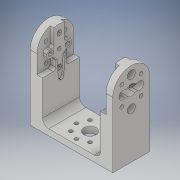
# Autodesk Inventor part: Module_Arm
Saved by Autodesk Inventor 2018 (Build 220112000, 112)
## iProperties
Created: 2016-10-25
Part Number: Module_Arm
Material: Generic
Document SubType Name: Modeling
Designer: Lucas
Density: 1 g/cm^3
Appearance: Default
Author: Lucas
Autodesk Inventor part; units mm, degrees
ref_plane "YZ Plane" through (0, 0, 0) normal (1, 0, 0) x (0, 1, 0)
sketch "Sketch1" plane through (0, 0, 0) normal (0, 0, 1) x (1, 0, 0)
  line L0 (0, 0) -> (47, 0)
  line L1 (47, 0) -> (47, 63)
  line L2 (47, 63) -> (57, 63)
  line L3 (57, 63) -> (57, -5)
  line L4 (57, -5) -> (-10, -5)
  line L5 (-10, -5) -> (-10, 63)
  line L6 (-10, 63) -> (0, 63)
  line L7 (0, 63) -> (0, 0)
  dimension "d0" = 47
  dimension "d1" = 63
  dimension "d2" = 10
  dimension "d13" = 5
  dimension "d64" = 10
  constraints: 16 end point, 5 perpendicular, 2 point on line, 1 horizontal, 1 vertical
  measures "d0" distance of L0.start L0.end
  measures "d1" distance of L0.end L1.end
  measures "d2" distance of L1.end L2.end
  measures "d13" distance between parallel lines of L4 L0
  measures "d64" distance of L5.end L6.end
extrude "U_Profile" add sketch "Sketch1" along normal blind 30
sketch "Sketch2" plane through (57, -5, 0) normal (1, 0, 0) x (0, 0, -1)
  circle A0 centre (-15, 50.6) radius 1.5
  line L0 (-15, 55.5625) -> (-15, -8.8186) construction
  line L1 (-30, 0) -> (-30, 68) projected
  line L2 (0, 68) -> (0, 0) projected
  line L3 (0, 68) -> (-30, 68) projected
  point P0 (0, 5)
  dimension "d7" = 3
  dimension "d8" = 30
  dimension "d9" = 15
  dimension "d10" = 17.4
  constraints: 2 end point, 1 centre point, 1 point on line, 1 vertical
  measures "d7" diameter of A0
  measures "d8" distance between parallel lines of L1 L2
  measures "d9" distance between parallel lines of L0 L2
  measures "d10" distance from line of A0.centre L3
extrude "Shaft_Opening" cut sketch "Sketch2" against normal up to surface (67 mm away)
sketch "Sketch4" plane through (-10, -5, 0) normal (-1, 0, 0) x (0, 0, 1)
  circle A0 centre (15, 50.6) radius 5
  circle A1 centre (15, 50.6) radius 1.5 projected
  point P0 (0, 5)
  dimension "d18" = 10
  constraints: 1 centre point, 1 concentric
  measures "d18" diameter of A0
extrude "Nut_Slot" cut sketch "Sketch4" against normal blind 5.5
sketch "Sketch6" plane through (0, 0, 0) normal (0, 1, 0) x (1, 0, 0)
  circle A0 centre (23.5, -15) radius 11 construction
  line L0 (0, -15) -> (46.0375, -15)
  line L1 (47, -30) -> (0, -30) projected
  line L2 (0, 0) -> (47, 0) projected
  line L3 (0, 0) -> (0, -30) projected
  line L4 (47, 0) -> (47, -30) projected
  circle A1 centre (12.5, -15) radius 1.5
  circle A2 centre (34.5, -15) radius 1.5
  line L5 (9.9716, -1.4716) -> (37.7642, -29.2642) construction
  line L6 (9.808, -28.692) -> (35.7154, -2.7846) construction
  line L7 (23.5, 2.3185) -> (23.5, -31.0285) construction
  circle A3 centre (15.7218, -7.2218) radius 1.5
  circle A4 centre (23.5, -4) radius 1.5
  circle A5 centre (31.2782, -7.2218) radius 1.5
  circle A6 centre (23.5, -26) radius 1.5
  circle A7 centre (15.7218, -22.7782) radius 1.5
  circle A8 centre (31.2782, -22.7782) radius 1.5
  dimension "d21" = 22
  dimension "d22" = 30
  dimension "d23" = 15
  dimension "d24" = 23.5
  dimension "d25" = 47
  dimension "d26" = 3
  dimension "d27" = 3
  dimension "d28" = 45
  dimension "d29" = 45
  dimension "d30" = 90
  dimension "d31" = 3
  dimension "d32" = 3
  dimension "d33" = 3
  dimension "d34" = 3
  dimension "d35" = 3
  dimension "d36" = 3
  constraints: 12 point on line, 8 centre point, 8 end point, 1 horizontal, 10 other
  measures "d22" distance between parallel lines of L1 L2
  measures "d23" distance between parallel lines of L2 L0
  measures "d24" distance from line of point (23.5, -15) L3
  measures "d25" distance between parallel lines of L4 L3
  measures "d26" diameter of A1
  measures "d27" diameter of A2
  measures "d28" angle of L5 L0
  measures "d29" angle of L0 L6
  measures "d30" angle of L0 L7
  measures "d31" diameter of A3
  measures "d32" diameter of A4
  measures "d33" diameter of A5
  measures "d34" diameter of A6
  measures "d35" diameter of A7
  measures "d36" diameter of A8
extrude "Docking_Holes_Front" cut sketch "Sketch6" against normal up to surface (5 mm away) contours A1 L0 | L0 A1 | A2 L0 | L0 A2 | A3 | A4 | A5 | A6 | A7 | A8
sketch "Sketch8" plane through (47, 0, 4) normal (-1, 0, 0) x (0, 0, 1)
  line L0 (19.4554, 45.6) -> (2.5446, 45.6) construction
  line L1 (11, 58.3863) -> (11, 17.922) construction
  line L2 (13, 24.6021) -> (9, 24.6021) construction
  line L3 (14.5, 43.6) -> (12.9998, 24.6)
  line L4 (7.5, 43.6) -> (9, 24.6021)
  line L5 (19.4554, 45.6) -> (13.9554, 45.6) construction
  line L6 (2.5446, 45.6) -> (8.0446, 45.6) construction
  line L7 (13, 58.6) -> (9, 58.6) construction
  line L8 (13.9554, 45.6) -> (12.7795, 61.6) construction
  line L9 (8.0446, 45.6) -> (9.2205, 61.6) construction
  line L10 (12.7795, 61.6) -> (9.2205, 61.6) construction
  line L11 (12.9998, 24.6) -> (9, 24.6021)
  line L12 (7.5, 43.6) -> (-4, 43.6)
  line L13 (14.5, 43.6) -> (26, 43.6)
  line L14 (-4, 0) -> (-4, 63) projected
  line L15 (-4, 43.6) -> (-4, 63)
  line L16 (-4, 63) -> (26, 63) projected
  line L17 (-4, 63) -> (26, 63)
  line L18 (26, 63) -> (26, 43.6)
  point P0 (11, 45.6)
  dimension "d48" = 4
  dimension "d52" = 19
  dimension "d54" = 5.5
  dimension "d55" = 5.5
  dimension "d56" = 4
  dimension "d57" = 13
  dimension "d58" = 16
  dimension "d59" = 16
  dimension "d109" = 2
  dimension "d183" = 2
  dimension "d189" = 3.9998
  dimension "d221" = 2
  dimension "d256" = 15
  dimension "d257" = 3.5
  constraints: 34 end point, 7 point on line, 4 horizontal, 2 collinear, 2 symmetric about line, 1 midpoint, 1 parallel, 1 perpendicular, 1 vertical, 1 other
  measures "d48" distance of L2.start L2.end
  measures "d52" vertical distance of L3.start L3.end
  measures "d54" distance of L0.start L5.end
  measures "d55" distance of L0.end L6.end
  measures "d56" distance of L7.start L7.end
  measures "d57" distance between parallel lines of L0 L7
  measures "d58" vertical distance of L5.end L8.end
  measures "d59" vertical distance of L6.end L9.end
  measures "d109" distance from line of L1 L4.end
  measures "d183" distance between parallel lines of L13 L0
  measures "d189" distance of L3.end L4.end
  measures "d221" distance from line of L12 point (11, 45.6)
  measures "d256" distance between parallel lines of L15 L1
  measures "d257" distance from line of L4.start L1
extrude "Servo_Horn_Slot" cut sketch "Sketch8" against normal blind 1.5
fillet "Fillet4" radius 2 2 edges at (47.75, 24.6021, 13) (47.75, 24.6, 16.9998)
fillet "Fillet9" radius 15 4 edges at (-5, 63, 0) (-5, 63, 30) (52.75, 63, 0) (52.75, 63, 30)
sketch "Sketch11" plane through (-10, -5, 0) normal (-1, 0, 0) x (0, 0, 1)
  circle A0 centre (15, 50.6) radius 11 construction
  circle A1 centre (15, 50.6) radius 1.5 projected
  line L0 (1.3636, 36.9636) -> (45.6005, 81.2005) construction
  line L1 (1.3398, 64.2602) -> (31.9798, 33.6202) construction
  line L2 (15, 20.4128) -> (15, 77.5107)
  circle A2 centre (7.2218, 42.8218) radius 1.5
  circle A3 centre (7.2218, 58.3782) radius 1.5
  circle A4 centre (22.7782, 42.8218) radius 1.5
  circle A5 centre (22.7782, 58.3782) radius 1.5
  point P0 (0, 5)
  dimension "d98" = 22
  dimension "d99" = 45
  dimension "d100" = 45
  dimension "d101" = 3
  dimension "d102" = 3
  dimension "d103" = 3
  dimension "d104" = 3
  constraints: 7 point on line, 6 end point, 5 centre point, 4 point on circle, 1 concentric, 1 vertical
  measures "d98" diameter of A0
  measures "d99" angle of L2 L0
  measures "d100" angle of L2 L1
  measures "d101" diameter of A2
  measures "d102" diameter of A3
  measures "d103" diameter of A4
  measures "d104" diameter of A5
extrude "Docking_Holes_Lateral" cut sketch "Sketch11" against normal up to surface (67 mm away) contours A2 | A3 | A4 | A5
ref_plane "Work Plane6" through (23.5, 0, 30) normal (1, 0, 0) x (0, 0, -1)
mirror "Mirror7" about plane through (23.5, 0, 30) normal (1, 0, 0) of "Servo_Horn_Slot", "Fillet4"
sketch "Sketch12" plane through (-10, -5, 0) normal (0, -1, 0) x (1, 0, 0)
  circle A0 centre (33.5, 15) radius 5
  line L0 (0, 0) -> (0, 30) projected
  line L1 (67, 0) -> (67, 30) projected
  line L2 (67, 0) -> (0, 0) projected
  line L3 (0, 30) -> (67, 30) projected
  point P0 (10, 0)
  dimension "d113" = 10
  dimension "d114" = 67
  dimension "d115" = 33.5
  dimension "d116" = 30
  dimension "d117" = 15
  constraints: 1 centre point
  measures "d113" diameter of A0
  measures "d114" distance between parallel lines of L0 L1
  measures "d115" distance from line of A0.centre L1
  measures "d116" distance between parallel lines of L2 L3
  measures "d117" distance from line of L3 A0.centre
extrude "Cable_Opening_Front" cut sketch "Sketch12" against normal up to surface (5 mm away) contours A0
sketch "Sketch13" plane through (-10, -5, 0) normal (-1, 0, 0) x (0, 0, 1)
  line L0 (13.5, 35.6) -> (16.5, 35.6)
  line L1 (16.5, 35.6) -> (16.5, 39.6)
  line L2 (16.5, 39.6) -> (13.5, 39.6)
  line L3 (13.5, 39.6) -> (13.5, 35.6)
  line L4 (15, -15.875) -> (15, 92.075) construction
  line L5 (0, 0) -> (0, 53) projected
  line L6 (30, 53) -> (30, 0) projected
  line L7 (-11.1125, 50.6) -> (45.1198, 50.6) construction
  circle A0 centre (7.2218, 58.3782) radius 1.5 projected
  circle A1 centre (7.2218, 42.8218) radius 1.5 projected
  line L8 (3.7218, 37.6) -> (29.75, 37.6) construction
  line L9 (10.2303, 49.1) -> (6.2303, 49.1)
  line L10 (6.2303, 49.1) -> (6.2303, 52.1)
  line L11 (6.2303, 52.1) -> (10.2303, 52.1)
  line L12 (10.2303, 52.1) -> (10.2303, 49.1)
  line L13 (8.2303, 31.9316) -> (8.2303, 57.3316) construction
  line L14 (13.5, 59.6) -> (16.5, 59.6)
  line L15 (16.5, 59.6) -> (16.5, 63.6)
  line L16 (16.5, 63.6) -> (13.5, 63.6)
  line L17 (13.5, 63.6) -> (13.5, 59.6)
  line L18 (-3.175, 61.6) -> (37.2514, 61.6) construction
  line L19 (19.7697, 49.1) -> (23.7697, 49.1)
  line L20 (23.7697, 49.1) -> (23.7697, 52.1)
  line L21 (23.7697, 52.1) -> (19.7697, 52.1)
  line L22 (19.7697, 52.1) -> (19.7697, 49.1)
  line L23 (21.7697, 37) -> (21.7697, 59.3316) construction
  circle A2 centre (15, 50.6) radius 5 projected
  dimension "d120" = 3
  dimension "d121" = 4
  dimension "d122" = 30
  dimension "d123" = 15
  dimension "d124" = 15.5564
  dimension "d125" = 7.7782
  dimension "d127" = 13
  dimension "d128" = 3
  dimension "d131" = 4
  dimension "d132" = 3
  dimension "d133" = 4
  dimension "d134" = 11
  dimension "d135" = 3
  dimension "d136" = 4
  constraints: 44 end point, 8 parallel, 6 horizontal, 4 perpendicular, 2 point on circle, 2 vertical, 1 collinear, 7 other
  measures "d120" distance of L2.end L1.end
  measures "d121" distance of L1.end L0.end
  measures "d122" distance between parallel lines of L5 L6
  measures "d123" distance between parallel lines of L5 L4
  measures "d124" distance of A0.centre A1.centre
  measures "d125" distance from line of A0.centre L7
  measures "d127" distance between parallel lines of L7 L8
  measures "d128" distance of L9.end L10.end
  measures "d131" distance of L10.end L11.end
  measures "d132" distance of L15.end L16.end
  measures "d133" distance of L16.end L14.start
  measures "d134" distance between parallel lines of L18 L7
  measures "d135" distance of L21.end L19.start
  measures "d136" distance of L20.end L21.end
extrude "Openings_ServoHorn_Fixation" cut sketch "Sketch13" against normal up to surface (10 mm away) contours L3 L2 L1 L0 | A2 L12 | L9 L10 L11 A2 | A2 L21 L20 L19 | L22 A2 | L17 L16 L15 L14
mirror "Mirror8" about plane through (23.5, 0, 30) normal (1, 0, 0) of "Openings_ServoHorn_Fixation"
fillet "Fillet11" radius 5 2 edges at (47, 0, 15) (0, 0, 15)
sketch "Sketch15" plane through (47, 43.6, 18.5) normal (-1, 0, 0) x (0, 0, 1)
  circle A0 centre (4.2782, -5.7782) radius 3.5 construction
  circle A1 centre (-11.2782, -5.7782) radius 3.5 construction
  circle A2 centre (4.2782, -5.7782) radius 1.5 projected
  circle A3 centre (-11.2782, -5.7782) radius 1.5 projected
  line L0 (-18.5, -38.6) -> (-18.5, 0) projected
  line L1 (-12.2697, 3.5) -> (-8.2697, 3.5) projected
  line L2 (11.5, -48.6) -> (11.5, 4.4) projected
  line L3 (11.5, 4.4) -> (11.5, -38.6) projected
  line L4 (11.5, -1.2782) -> (0.7782, -1.2782)
  line L5 (0.7782, -1.2782) -> (0.7782, -10.2782)
  line L6 (0.7782, -10.2782) -> (11.5, -10.2782)
  line L7 (11.5, -10.2782) -> (11.5, -1.2782)
  line L8 (-18.5, -0.7782) -> (-7.7782, -0.7782)
  line L9 (-7.7782, -0.7782) -> (-7.7782, -10.7782)
  line L10 (-7.7782, -10.7782) -> (-18.5, -10.7782)
  line L11 (-18.5, -10.7782) -> (-18.5, -0.7782)
  point P0 (-18.5, -43.6)
  point P1 (11.5, 0)
  point P2 (-18.5, 4.4)
  dimension "d153" = 7
  dimension "d154" = 7
  dimension "d199" = 9
  dimension "d200" = 4.5
  dimension "d201" = 10
  dimension "d202" = 5
  constraints: 16 end point, 4 parallel, 2 centre point, 2 concentric, 2 horizontal, 2 perpendicular, 2 point on line, 2 tangent
  measures "d153" diameter of A0
  measures "d154" diameter of A1
  measures "d199" distance between parallel lines of L6 L4
  measures "d200" distance from line of A0.centre L4
  measures "d201" distance of L10.end L8.start
  measures "d202" distance from line of A1.centre L8
extrude "Nut_Slot_Docking_Lateral_01" cut sketch "Sketch15" against normal blind 4.5
sketch "Sketch16" plane through (48.5, 0, 4) normal (-1, 0, 0) x (0, 0, 1)
  circle A0 centre (18.7782, 53.3782) radius 1.5 projected
  circle A1 centre (3.2218, 53.3782) radius 1.5 projected
  arc A2 (26, 48) -> (-4, 48) centre (11, 48) ccw projected
  line L0 (26, 62.377) -> (15.2782, 62.377)
  line L1 (15.2782, 62.377) -> (15.2782, 48.3782)
  line L2 (15.2782, 48.3782) -> (26, 48.3782)
  line L3 (26, 48.3782) -> (26, 62.377)
  line L4 (26, 48) -> (26, 43.6) projected
  line L5 (6.7218, 62.377) -> (-4, 62.377)
  line L6 (-4, 62.377) -> (-4, 48.3782)
  line L7 (-4, 48.3782) -> (6.7218, 48.3782)
  line L8 (6.7218, 48.3782) -> (6.7218, 62.377)
  line L9 (-4, 43.6) -> (-4, 48) projected
  point P0 (-4, 0)
  dimension "d205" = 3.5
  dimension "d208" = 3.5
  dimension "d210" = 5
  dimension "d211" = 5
  constraints: 16 end point, 4 parallel, 2 collinear, 2 horizontal, 2 perpendicular, 2 point on circle
  measures "d205" distance from line of A0.centre L1
  measures "d208" distance from line of L8 A1.centre
  measures "d210" distance from line of L2 A0.centre
  measures "d211" distance from line of L7 A1.centre
extrude "Nut_Slot_Docking_Lateral_02" cut sketch "Sketch16" against normal blind 3
mirror "Mirror10" about plane through (23.5, 0, 30) normal (1, 0, 0) of "Nut_Slot_Docking_Lateral_01", "Nut_Slot_Docking_Lateral_02"
sketch "Sketch17" plane through (57, -5, 30) normal (1, 0, 0) x (0, 0, -1)
  circle A0 centre (21.7697, 50.6) radius 3.25
  circle A1 centre (8.2303, 50.6) radius 3.25
  circle A2 centre (15, 61.6) radius 3.25
  line L0 (34.925, 50.6) -> (-15.875, 50.6) construction
  line L1 (10.2303, 49.1) -> (6.2303, 49.1) projected
  line L2 (6.2303, 52.1) -> (10.2303, 52.1) projected
  line L3 (15, 16.4203) -> (15, 83.0987) construction
  line L4 (13.5, 35.6) -> (13.5, 39.6) projected
  line L5 (16.5, 39.6) -> (16.5, 35.6) projected
  line L6 (16.5, 35.6) -> (13.5, 35.6) projected
  line L7 (13.5, 39.6) -> (16.5, 39.6) projected
  line L8 (13.5, 63.6) -> (16.5, 63.6) projected
  line L9 (16.5, 59.6) -> (13.5, 59.6) projected
  line L10 (6.2303, 49.1) -> (6.2303, 52.1) projected
  line L11 (10.2303, 49.1) -> (10.2303, 52.1) projected
  line L12 (23.7697, 52.1) -> (23.7697, 49.1) projected
  line L13 (16.5, 39.6) -> (13.5, 35.6) construction
  line L14 (13.5, 35.6) -> (13.5, 39.6) projected
  line L15 (13.5, 39.6) -> (16.5, 35.6) construction
  circle A3 centre (15, 37.6) radius 3.25
  line L16 (19.7697, 49.1) -> (19.7697, 52.1) projected
  point P0 (30, 5)
  dimension "d163" = 6.5
  dimension "d164" = 6.5
  dimension "d165" = 6.5
  dimension "d166" = 3
  dimension "d167" = 1.5
  dimension "d168" = 3
  dimension "d169" = 1.5
  dimension "d170" = 4
  dimension "d172" = 4
  dimension "d173" = 2
  dimension "d174" = 4
  dimension "d175" = 2
  dimension "d190" = 11
  dimension "d192" = 6.5
  dimension "d254" = 4
  dimension "d255" = 2
  constraints: 8 end point, 4 centre point, 3 point on line, 1 coincident, 1 midpoint, 1 vertical
  measures "d163" diameter of A0
  measures "d164" diameter of A1
  measures "d165" diameter of A2
  measures "d166" distance between parallel lines of L1 L2
  measures "d167" distance between parallel lines of L2 L0
  measures "d168" distance between parallel lines of L4 L5
  measures "d169" distance between parallel lines of L4 L3
  measures "d170" distance between parallel lines of L6 L7
  measures "d172" distance between parallel lines of L8 L9
  measures "d173" distance from line of L8 A2.centre
  measures "d174" distance between parallel lines of L10 L11
  measures "d175" distance from line of L11 A1.centre
  measures "d190" distance from line of L0 A2.centre
  measures "d192" diameter of A3
  measures "d254" distance between parallel lines of L16 L12
  measures "d255" distance from line of A0.centre L12
extrude "Servo_Screws_Slots" cut sketch "Sketch17" against normal blind 5
mirror "Mirror11" about plane through (23.5, 0, 30) normal (1, 0, 0) of "Servo_Screws_Slots"
fillet "Fillet12" radius 1 16 edges at (50.25, 30.6, 16.5) (50.25, 34.6, 16.5) (50.25, 34.6, 13.5) (50.25, 30.6, 13.5) (50.25, 44.1, 19.7697) (50.25, 44.1, 23.7697) (50.25, 47.1, 23.7697) (50.25, 47.1, 19.7697) (50.25, 58.6, 13.5) (50.25, 58.6, 16.5) (50.25, 47.1, 10.2303) (50.25, 54.6, 16.5) (50.25, 54.6, 13.5) (50.25, 44.1, 6.2303) (50.25, 47.1, 6.2303) (50.25, 44.1, 10.2303)
mirror "Mirror12" about plane through (23.5, 0, 30) normal (1, 0, 0) of "Fillet12"
fillet "Fillet13" radius 2 6 edges at (50, 48.3782, 19.2782) (49.25, 42.3218, 19.2782) (49.25, 33.3218, 19.2782) (49.25, 32.8218, 10.7218) (49.25, 42.8218, 10.7218) (50, 48.3782, 10.7218)
fillet "Fillet14" radius 2 6 edges at (-2.25, 33.3218, 19.2782) (-2.25, 42.3218, 19.2782) (-3, 48.3782, 19.2782) (-3, 48.3782, 10.7218) (-2.25, 32.8218, 10.7218) (-2.25, 42.8218, 10.7218)
sketch "Sketch22" plane through (57, -5, 30) normal (1, 0, 0) x (0, 0, -1)
  line L0 (7.5, 27) -> (22.5, 27)
  line L1 (22.5, 27) -> (22.5, 10)
  line L2 (22.5, 10) -> (7.5, 10)
  line L3 (7.5, 10) -> (7.5, 27)
  line L4 (30, 0) -> (0, 0) projected
  line L5 (15, 75.1344) -> (15, -33.1284) construction
  line L6 (30, 53) -> (30, 0) projected
  line L7 (0, 0) -> (0, 53) projected
  point P0 (30, 5)
  dimension "d228" = 10
  dimension "d229" = 17
  dimension "d230" = 15
  dimension "d231" = 30
  dimension "d232" = 15
  constraints: 10 end point, 2 parallel, 1 horizontal, 1 perpendicular, 1 vertical, 1 other
  measures "d228" distance between parallel lines of L4 L2
  measures "d229" distance of L0.end L1.end
  measures "d230" distance between parallel lines of L3 L1
  measures "d231" distance between parallel lines of L6 L7
  measures "d232" distance from line of point (30, 5) L5
extrude "Extrusion21" [suppressed]
fillet "Fillet16" [suppressed]
sketch "Sketch23" plane through (47, 43.6, 18.5) normal (-1, 0, 0) x (0, 0, 1)
  line L0 (-18.5, -2.7782) -> (11.5, -2.7782)
  line L1 (11.5, -2.7782) -> (11.5, 0)
  line L2 (11.5, 0) -> (-18.5, 0)
  line L3 (-18.5, 0) -> (-18.5, -2.7782)
  line L4 (11.5, 0) -> (0, 0) projected
  line L5 (11.5, 0) -> (11.5, -1.2782) projected
  line L6 (-18.5, -0.7782) -> (-18.5, 0) projected
  line L7 (-18.5, -0.7782) -> (-9.7782, -0.7782) projected
  point P0 (-18.5, -43.6)
  dimension "d241" = 2
  constraints: 8 end point, 3 collinear, 2 parallel, 1 horizontal, 1 perpendicular
  measures "d241" distance between parallel lines of L7 L0
extrude "Material_Reduction_01" cut sketch "Sketch23" against normal up to surface (1.5 mm away)
sketch "Sketch24" plane through (57, -5, 30) normal (1, 0, 0) x (0, 0, -1)
  circle A0 centre (15, 50.8) radius 4.25
  line L0 (15, -22.1692) -> (15, 79.8112) construction
  line L1 (30, 53) -> (30, 0) projected
  line L2 (0, 0) -> (0, 53) projected
  circle A1 centre (15, 50.6) radius 1.5 projected
  point P0 (30, 5)
  dimension "d242" = 8.5
  dimension "d243" = 30
  dimension "d244" = 15
  dimension "d245" = 0.2
  constraints: 2 end point, 1 centre point, 1 point on line, 1 vertical
  measures "d242" diameter of A0
  measures "d243" distance between parallel lines of L1 L2
  measures "d244" distance between parallel lines of L0 L2
  measures "d245" distance of A0.centre A1.centre
extrude "Servo_Horn_Opening" cut sketch "Sketch24" against normal up to surface (10 mm away)
mirror "Mirror13" about plane through (23.5, 0, 30) normal (1, 0, 0) of "Material_Reduction_01"
sketch "Sketch25" plane through (48.5, 0, 4) normal (-1, 0, 0) x (0, 0, 1)
  line L0 (17.2782, 42.3218) -> (26, 42.3218) projected
  line L1 (25.9952, 48.3782) -> (17.2782, 48.3782) projected
  line L2 (26, 42.3218) -> (21, 42.3218)
  line L3 (21, 42.3218) -> (21, 48.3782)
  line L4 (21, 48.3782) -> (26, 48.3782)
  line L5 (26, 48.3782) -> (26, 42.3218)
  circle A0 centre (11, 45.8) radius 4.25 projected
  line L6 (4.7218, 48.3782) -> (-3.9952, 48.3782) projected
  line L7 (-4, 42.8218) -> (1, 42.8218)
  line L8 (1, 42.8218) -> (1, 48.3782)
  line L9 (1, 48.3782) -> (-4, 48.3782)
  line L10 (-4, 48.3782) -> (-4, 42.8218)
  point P0 (-4, 0)
  dimension "d248" = 10
  dimension "d252" = 10
  constraints: 16 end point, 4 parallel, 2 horizontal, 2 perpendicular, 2 point on line
  measures "d248" distance from line of A0.centre L3
  measures "d252" distance from line of L8 A0.centre
extrude "Material_Reduction_02" cut sketch "Sketch25" against normal up to surface (3 mm away) contours L3 L1 L4 L5 L0 | L8 L7 L10 L9 L6
fillet "Fillet17" radius 2 4 edges at (50, 42.3218, 25) (50, 48.3782, 25) (50, 48.3782, 5) (50, 42.8218, 5)
ref_plane "Work Plane8" through (0, 0, 15) normal (0, 0, 1) x (1, 0, 0)
mirror "Mirror14" about plane through (23.5, 0, 30) normal (1, 0, 0) of "Material_Reduction_02"
mirror "Mirror15" about plane through (23.5, 0, 30) normal (1, 0, 0) of "Fillet17"
fillet "Fillet18" radius 2 8 edges at (54.5, 44.091, 18.8913) (54.5, 44.091, 11.1087) (54.5, 47.2763, 18.9854) (54.5, 47.2763, 11.0146) (-7.5, 47.8775, 19.4512) (-7.5, 47.8775, 10.5488) (-7.5, 43.3225, 19.4512) (-7.5, 43.3225, 10.5488)
equation "\"d64\" = d2"
equation "\"d9\" = 0.5 * d8"
equation "\"d23\" = 0.5 * d22"
equation "\"d24\" = 0.5 * d25"
body "Solid1"
